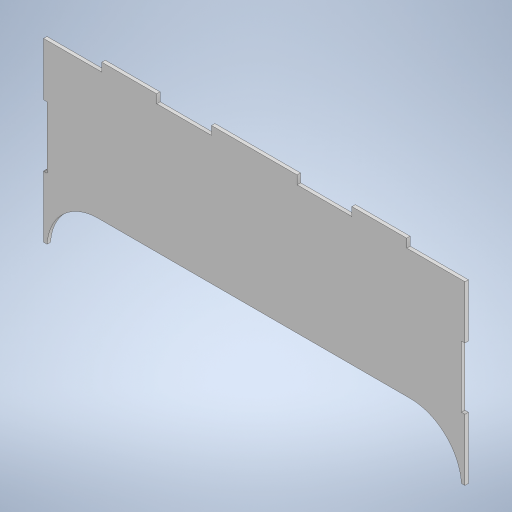
# Autodesk Inventor part: front
Saved by Autodesk Inventor 2023 (Build 270158000, 158)
## iProperties
Created: 2023-04-26
Part Number: front
Material: Generic
Document SubType Name: Modeling
Designer: Unnar
Density: 1 g/cm^3
Appearance: Default
Author: Unnar
Autodesk Inventor part; units mm, degrees
ref_plane "YZ Plane" through (0, 0, 0) normal (1, 0, 0) x (0, 1, 0)
ref_plane "XZ Plane" through (0, 0, 0) normal (0, 1, 0) x (-1, 0, 0)
ref_plane "XY Plane" through (0, 0, 0) normal (0, 0, 1) x (1, 0, 0)
sketch "Sketch1" plane through (0, 0, 0) normal (0, 0, 1) x (1, 0, 0)
  line L0 (-146.6185, 70.3133) -> (95.3815, 70.3133)
  line L1 (95.3815, 70.3133) -> (95.3815, -9.6867)
  line L2 (2.9423, -9.6867) -> (-45.2664, -9.6867)
  line L3 (-146.6185, -9.6867) -> (-146.6185, 70.3133)
  line L4 (-116.6185, -9.6867) -> (-45.2664, -9.6867)
  line L5 (65.3815, -9.6867) -> (2.9423, -9.6867)
  arc A0 (-116.6185, -9.6867) -> (-146.6185, -39.6867) centre (-116.6185, -39.6867) ccw
  arc A1 (95.3815, -39.6867) -> (65.3815, -9.6867) centre (65.3815, -39.6867) ccw
  line L6 (-146.6185, -9.6867) -> (-146.6185, -39.6867)
  line L7 (95.3815, -9.6867) -> (95.3815, -39.6867)
  point P0 (0, 0)
  dimension "d0" = 242
  dimension "d1" = 80
  dimension "d2" = 30
  constraints: 16 end point, 4 point on circle, 4 tangent, 3 horizontal, 3 parallel, 2 centre point, 2 point on line, 1 equal radius, 1 perpendicular, 1 vertical
  measures "d0" distance of L0.start L0.end
  measures "d1" distance of L0.end L1.end
  measures "d2" radius of A0
extrude "Extrusion1" add sketch "Sketch1" along normal blind 2
sketch "Sketch2" plane through (0, 0, 2) normal (0, 0, 1) x (1, 0, 0)
  line L0 (95.3815, 70.3133) -> (-146.6185, 70.3133) projected
  line L1 (-146.6185, 70.3133) -> (-114.6185, 70.3133)
  line L2 (-114.6185, 70.3133) -> (-114.6185, 65.3133)
  line L3 (-114.6185, 65.3133) -> (-146.6185, 65.3133)
  line L4 (-146.6185, 65.3133) -> (-146.6185, 70.3133)
  line L5 (-82.6185, 70.3133) -> (-50.6185, 70.3133)
  line L6 (-50.6185, 70.3133) -> (-50.6185, 65.3133)
  line L7 (-50.6185, 65.3133) -> (-82.6185, 65.3133)
  line L8 (-82.6185, 65.3133) -> (-82.6185, 70.3133)
  line L9 (-0.6185, 70.3133) -> (31.3815, 70.3133)
  line L10 (31.3815, 70.3133) -> (31.3815, 65.3133)
  line L11 (31.3815, 65.3133) -> (-0.6185, 65.3133)
  line L12 (-0.6185, 65.3133) -> (-0.6185, 70.3133)
  line L13 (95.3815, -39.6867) -> (95.3815, 70.3133) projected
  line L14 (95.3815, 70.3133) -> (63.3815, 70.3133)
  line L15 (63.3815, 70.3133) -> (63.3815, 65.3133)
  line L16 (63.3815, 65.3133) -> (95.3815, 65.3133)
  line L17 (95.3815, 65.3133) -> (95.3815, 70.3133)
  point P0 (0, 0)
  dimension "d5" = 32
  dimension "d6" = 32
  dimension "d7" = 32
  dimension "d8" = 32
  dimension "d9" = 32
  dimension "d10" = 32
  dimension "d11" = 50
  dimension "d12" = 5
  constraints: 32 end point, 8 parallel, 5 point on line, 4 horizontal, 4 perpendicular
  measures "d5" distance of L2.end L3.end
  measures "d6" distance between parallel lines of L8 L2
  measures "d7" distance of L6.end L7.end
  measures "d8" distance of L15.end L16.end
  measures "d9" distance between parallel lines of L10 L15
  measures "d10" distance of L10.end L11.end
  measures "d11" distance between parallel lines of L12 L6
  measures "d12" distance of L3.end L0.end
extrude "Extrusion2" cut sketch "Sketch2" against normal blind 2
sketch "Sketch3" plane through (0, 0, 2) normal (0, 0, 1) x (1, 0, 0)
  line L0 (-146.6185, 65.3133) -> (-146.6185, -39.6867) projected
  line L1 (-146.6185, 65.3133) -> (-148.6185, 65.3133)
  line L2 (-148.6185, 65.3133) -> (-148.6185, 34.3133)
  line L3 (-148.6185, 34.3133) -> (-146.6185, 34.3133)
  line L4 (-146.6185, 34.3133) -> (-146.6185, 65.3133)
  line L5 (-146.6185, -1.6867) -> (-148.6185, -1.6867)
  line L6 (-148.6185, -1.6867) -> (-148.6185, -37.6867)
  line L7 (-146.6185, -37.6867) -> (-146.6185, -1.6867)
  line L8 (95.3815, -39.6867) -> (95.3815, 65.3133) projected
  line L9 (95.3815, 65.3133) -> (97.3815, 65.3133)
  line L10 (97.3815, 65.3133) -> (97.3815, 34.3133)
  line L11 (97.3815, 34.3133) -> (95.3815, 34.3133)
  line L12 (95.3815, 34.3133) -> (95.3815, 65.3133)
  line L13 (95.3815, -1.6867) -> (97.3815, -1.6867)
  line L14 (97.3815, -1.6867) -> (97.3815, -37.6867)
  line L15 (95.3815, -37.6867) -> (95.3815, -1.6867)
  line L16 (-148.6185, -37.6867) -> (-146.6185, -37.6867)
  line L17 (95.3815, -39.6867) -> (95.3815, 65.3133) projected
  line L18 (95.3815, -37.6867) -> (97.3815, -37.6867)
  point P0 (-146.6185, -37.6867)
  point P1 (95.3815, -37.6867)
  dimension "d34" = 31
  dimension "d35" = 36
  dimension "d36" = 2
  dimension "d37" = 2
  dimension "d39" = 36
  dimension "d40" = 36
  constraints: 32 end point, 6 parallel, 6 point on line, 4 horizontal, 4 perpendicular
  measures "d34" distance of L1.end L2.end
  measures "d35" distance between parallel lines of L13 L11
  measures "d36" distance of L8.end L9.end
  measures "d37" distance of L0.start L1.end
  measures "d39" distance of L5.end L6.end
  measures "d40" distance of L13.end L14.end
extrude "Extrusion3" add sketch "Sketch3" against normal blind 2
sketch "Sketch4" plane through (0, 0, 2) normal (0, 0, 1) x (1, 0, 0)
  line L0 (-148.6185, -37.6867) -> (-146.6185, -37.6867) projected
  line L1 (-148.6185, -37.6867) -> (112.9742, -37.6867)
  line L2 (112.9742, -37.6867) -> (112.9742, -65.6367)
  line L3 (112.9742, -65.6367) -> (-148.6185, -65.6367)
  line L4 (-148.6185, -65.6367) -> (-148.6185, -37.6867)
  point P0 (0, 0)
  constraints: 8 end point, 2 parallel, 1 horizontal, 1 perpendicular
extrude "Extrusion4" cut sketch "Sketch4" against normal blind 2
body "Solid1"
